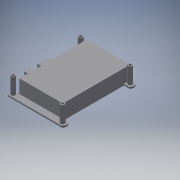
# Autodesk Inventor part: raspberry+touch
Saved by Autodesk Inventor 2019 (Build 230136000, 136)
## iProperties
Created: 2021-11-18
Part Number: raspberry+touch
Material: Generic
Document SubType Name: Modeling
Designer: Pokick
Density: 1 g/cm^3
Appearance: Default
Author: Pokick
Autodesk Inventor part; units mm, degrees
ref_plane "YZ Plane" through (0, 0, 0) normal (1, 0, 0) x (0, 1, 0)
ref_plane "XZ Plane" through (0, 0, 0) normal (0, 1, 0) x (-1, 0, 0)
ref_plane "XY Plane" through (0, 0, 0) normal (0, 0, 1) x (1, 0, 0)
sketch "Sketch1" plane through (0, 0, 0) normal (0, 1, 0) x (-1, 0, 0)
  line L0 (-29.02, 49.29) -> (29.02, 49.29)
  line L1 (29.02, 49.29) -> (29.02, 40.715) construction
  line L2 (29.02, -49.29) -> (-29.02, -49.29)
  line L3 (-29.02, -49.29) -> (-29.02, -40.715) construction
  line L4 (-29.02, 49.29) -> (29.02, -49.29) construction
  line L5 (29.02, 49.29) -> (-29.02, -49.29) construction
  line L6 (-33, 45) -> (33, 45) construction
  line L7 (33, 45) -> (33, -45) construction
  line L8 (33, -45) -> (-33, -45) construction
  line L9 (-33, -45) -> (-33, 45) construction
  line L10 (-33, 45) -> (33, -45) construction
  line L11 (33, 45) -> (-33, -45) construction
  circle A0 centre (33, 45) radius 1.5
  circle A1 centre (33, -45) radius 1.5
  circle A2 centre (-33, -45) radius 1.5
  circle A3 centre (-33, 45) radius 1.5
  line L12 (-38.27, 49.29) -> (38.27, 49.29) construction
  line L13 (38.27, 49.29) -> (38.27, -49.29) construction
  line L14 (38.27, -49.29) -> (-38.27, -49.29) construction
  line L15 (-38.27, -49.29) -> (-38.27, 49.29) construction
  line L16 (-38.27, 49.29) -> (38.27, -49.29) construction
  line L17 (38.27, 49.29) -> (-38.27, -49.29) construction
  line L18 (-38.27, 40.715) -> (29.02, 40.715) construction
  line L19 (38.27, 40.715) -> (38.27, -40.715) construction
  line L20 (38.27, -40.715) -> (-38.27, -40.715) construction
  line L21 (-38.27, -40.715) -> (-38.27, 40.715) construction
  line L22 (-38.27, 40.715) -> (38.27, -40.715) construction
  line L23 (38.27, 40.715) -> (-38.27, -40.715) construction
  line L24 (29.02, 49.29) -> (36.02, 49.29)
  line L25 (29.02, 40.715) -> (36.02, 40.715)
  arc A4 (36.02, 40.715) -> (36.02, 49.29) centre (33.06, 45.0025) ccw
  line L26 (29.02, 40.715) -> (29.02, -40.715)
  line L27 (0, 49.29) -> (0, -49.29) construction
  line L28 (-29.02, 0) -> (29.02, 0) construction
  line L29 (-38.27, -49.29) -> (38.27, -49.29) construction
  line L30 (-38.27, -40.715) -> (38.27, -40.715) construction
  line L31 (29.02, -49.29) -> (36.02, -49.29)
  line L32 (29.02, -40.715) -> (36.02, -40.715)
  arc A5 (36.02, -49.29) -> (36.02, -40.715) centre (33.06, -45.0025) ccw
  line L33 (0, -49.29) -> (0, 49.29) construction
  line L34 (-33, 45) -> (-33, -45) construction
  line L35 (38.27, 49.29) -> (-38.27, 49.29) construction
  line L36 (-38.27, 49.29) -> (-38.27, -49.29) construction
  line L37 (-38.27, -49.29) -> (38.27, -49.29) construction
  line L38 (38.27, 40.715) -> (-38.27, 40.715) construction
  line L39 (-38.27, -40.715) -> (38.27, -40.715) construction
  line L40 (-29.02, 49.29) -> (-36.02, 49.29)
  line L41 (-29.02, 40.715) -> (-36.02, 40.715)
  arc A6 (-36.02, 49.29) -> (-36.02, 40.715) centre (-33.06, 45.0025) ccw
  line L42 (38.27, -49.29) -> (-38.27, -49.29) construction
  line L43 (-29.02, -49.29) -> (-36.02, -49.29)
  line L44 (38.27, -40.715) -> (-38.27, -40.715) construction
  line L45 (-29.02, -40.715) -> (-36.02, -40.715)
  arc A7 (-36.02, -40.715) -> (-36.02, -49.29) centre (-33.06, -45.0025) ccw
  line L46 (-29.02, -40.715) -> (-29.02, 40.715)
  line L47 (-29.02, 40.715) -> (-29.02, 49.29) construction
  line L48 (29.02, 40.715) -> (38.27, 40.715) construction
  line L49 (29.02, -40.715) -> (29.02, -49.29) construction
  point P0 (0, 0)
  dimension "d0" = 58.04
  dimension "d1" = 98.58
  dimension "d2" = 66
  dimension "d3" = 90
  dimension "d4" = 3
  dimension "d5" = 3
  dimension "d6" = 3
  dimension "d7" = 3
  dimension "d8" = 76.54
  dimension "d9" = 98.58
  dimension "d10" = 76.54
  dimension "d11" = 81.43
  dimension "d12" = 7
  dimension "d13" = 7
  constraints: 100 end point, 22 symmetric about line, 17 parallel, 13 point on line, 11 midpoint, 9 perpendicular, 8 centre point, 8 point on circle, 5 horizontal, 4 coincident, 1 tangent, 3 other
  measures "d0" distance of L2.start L2.end
  measures "d1" distance of L0.end L2.start
  measures "d2" distance of L7.end L8.end
  measures "d3" distance of L6.end L7.end
  measures "d4" diameter of A0
  measures "d5" diameter of A1
  measures "d6" diameter of A2
  measures "d7" diameter of A3
  measures "d8" distance of L13.end L14.end
  measures "d9" distance of L12.end L13.end
  measures "d10" distance of L19.end L20.end
  measures "d11" distance of L19.start L19.end
  measures "d12" distance of L0.end L24.end
  measures "d13" distance of L1.end L25.end
extrude "Extrusion1" add sketch "Sketch1" along normal blind 2
sketch "Sketch2" plane through (0, 2, 0) normal (0, 1, 0) x (1, 0, 0)
  line L0 (29.02, -49.29) -> (-29.02, -49.29) construction
  line L1 (-29.02, -49.29) -> (-29.02, 49.29) construction
  line L2 (-29.02, 49.29) -> (29.02, 49.29) construction
  line L3 (29.02, 49.29) -> (29.02, -49.29) construction
  line L4 (29.02, -49.29) -> (-29.02, 49.29) construction
  line L5 (-29.02, -49.29) -> (29.02, 49.29) construction
  line L6 (29.02, 40.715) -> (29.02, -40.715) projected
  line L7 (-29.02, 49.29) -> (29.02, 49.29)
  line L8 (29.02, 49.29) -> (29.02, -40.71)
  line L9 (29.02, -40.71) -> (-29.02, -40.71)
  line L10 (-29.02, -40.71) -> (-29.02, 49.29)
  point P0 (0, 0)
  dimension "d16" = 58.04
  dimension "d17" = 98.58
  dimension "d18" = 90
  constraints: 20 end point, 4 parallel, 2 horizontal, 2 midpoint, 2 perpendicular, 1 point on line
  measures "d16" distance of L1.end L2.end
  measures "d17" distance of L0.end L1.end
  measures "d18" distance of L7.end L8.end
extrude "Extrusion2" add sketch "Sketch2" along normal blind 18
sketch "Sketch3" plane through (-29.02, 0, -40.715) normal (-1, 0, 0) x (0, 0, 1)
  line L0 (-8.575, 0) -> (-8.575, 2) projected
  line L1 (-8.575, 0) -> (37.425, 0) construction
  line L2 (81.43, 0) -> (0, 0) construction
  line L3 (37.425, 0) -> (52.425, 0) construction
  line L4 (37.425, 0) -> (52.425, 0)
  line L5 (52.425, 0) -> (52.425, 20)
  line L6 (52.425, 20) -> (37.425, 20)
  line L7 (37.425, 20) -> (37.425, 0)
  line L8 (81.43, 0) -> (90.005, 0) construction
  line L9 (90.005, 0) -> (70.005, 0) construction
  line L10 (70.005, 0) -> (62.005, 0) construction
  line L11 (62.005, 0) -> (70.005, 0)
  line L12 (70.005, 0) -> (70.005, 20)
  line L13 (70.005, 20) -> (62.005, 20)
  line L14 (62.005, 20) -> (62.005, 0)
  point P0 (40.715, 0)
  dimension "d21" = 46
  dimension "d22" = 15
  dimension "d23" = 20
  dimension "d24" = 15
  dimension "d25" = 20
  dimension "d26" = 8
  dimension "d27" = 8
  dimension "d28" = 20
  constraints: 24 end point, 4 parallel, 4 point on line, 2 horizontal, 2 perpendicular
  measures "d21" distance of L0.start L1.end
  measures "d22" distance of L1.end L3.end
  measures "d23" distance of L5.end L4.end
  measures "d24" distance between parallel lines of L7 L5
  measures "d25" distance of L8.end L9.end
  measures "d26" distance of L9.end L10.end
  measures "d27" distance of L13.end L12.end
  measures "d28" distance of L12.end L11.end
extrude "Extrusion3" add sketch "Sketch3" along normal blind 5
sketch "Sketch5" plane through (0, 0, 0) normal (0, -1, 0) x (1, 0, 0)
  circle A0 centre (-33, 45) radius 1.5 construction
  line L0 (33, -45) -> (-33, -45) construction
  line L1 (-33, -45) -> (-33, 45) construction
  line L2 (-33, 45) -> (33, 45) construction
  line L3 (33, 45) -> (33, -45) construction
  line L4 (33, -45) -> (-33, 45) construction
  line L5 (-33, -45) -> (33, 45) construction
  circle A1 centre (-33, -45) radius 1.5
  circle A2 centre (33, -45) radius 1.5
  circle A3 centre (33, 45) radius 1.5 projected
  circle A4 centre (33, 45) radius 1.5
  circle A5 centre (-33, 45) radius 1.5
  line L6 (-35.5, -43.5566) -> (-33, -42.1132)
  line L7 (-33, -42.1132) -> (-30.5, -43.5566)
  line L8 (-30.5, -43.5566) -> (-30.5, -46.4434)
  line L9 (-30.5, -46.4434) -> (-33, -47.8868)
  line L10 (-33, -47.8868) -> (-35.5, -46.4434)
  line L11 (-35.5, -46.4434) -> (-35.5, -43.5566)
  line L12 (30.5, -43.5566) -> (33, -42.1132)
  line L13 (33, -42.1132) -> (35.5, -43.5566)
  line L14 (35.5, -43.5566) -> (35.5, -46.4434)
  line L15 (35.5, -46.4434) -> (33, -47.8868)
  line L16 (33, -47.8868) -> (30.5, -46.4434)
  line L17 (30.5, -46.4434) -> (30.5, -43.5566)
  line L18 (30.5, 46.4434) -> (33, 47.8868)
  line L19 (33, 47.8868) -> (35.5, 46.4434)
  line L20 (35.5, 46.4434) -> (35.5, 43.5566)
  line L21 (35.5, 43.5566) -> (33, 42.1132)
  line L22 (33, 42.1132) -> (30.5, 43.5566)
  line L23 (30.5, 43.5566) -> (30.5, 46.4434)
  line L24 (-35.5, 46.4434) -> (-33, 47.8868)
  line L25 (-33, 47.8868) -> (-30.5, 46.4434)
  line L26 (-30.5, 46.4434) -> (-30.5, 43.5566)
  line L27 (-30.5, 43.5566) -> (-33, 42.1132)
  line L28 (-33, 42.1132) -> (-35.5, 43.5566)
  line L29 (-35.5, 43.5566) -> (-35.5, 46.4434)
  point P0 (0, 0)
  point P1 (30.5, 45)
  point P2 (-35.5, 45)
  dimension "d31" = 3
  dimension "d32" = 3
  dimension "d33" = 3
  dimension "d34" = 3
  dimension "d35" = 5
  dimension "d36" = 5
  dimension "d37" = 5
  dimension "d38" = 5
  constraints: 60 end point, 8 coincident, 4 centre point, 4 midpoint, 4 parallel, 2 point on line, 1 horizontal, 1 perpendicular, 52 other
  measures "d31" diameter of A1
  measures "d32" diameter of A2
  measures "d33" diameter of A4
  measures "d34" diameter of A5
  measures "d35" distance between parallel lines of L26 L29
  measures "d36" distance between parallel lines of L8 L11
  measures "d37" distance between parallel lines of L17 L14
  measures "d38" distance between parallel lines of L23 L20
extrude "Extrusion4" add sketch "Sketch5" against normal blind 22 from surface at -2
sketch "Sketch6" plane through (0, 0, 0) normal (0, -1, 0) x (1, 0, 0)
  line L0 (-35.8509, -30.6551) -> (-35.8509, -21.9955) construction
  line L1 (-35.8509, -21.9955) -> (-14.7214, -21.9955) construction
  line L2 (-14.7214, -21.9955) -> (-14.7214, -30.6551) construction
  line L3 (-14.7214, -30.6551) -> (-35.8509, -30.6551) construction
  point P0 (0, 0)
  constraints: 2 other
sketch "Sketch7" plane through (36.02, 0, -49.29) normal (0, 0, -1) x (-1, 0, 0)
  line L0 (36.02, 0) -> (63.02, 0) construction
  line L1 (0, 0) -> (72.04, 0) projected
  line L2 (63.02, 0) -> (11.02, 0)
  line L3 (11.02, 0) -> (11.02, 16)
  line L4 (11.02, 16) -> (63.02, 16)
  line L5 (63.02, 16) -> (63.02, 0)
  dimension "d41" = 27
  dimension "d42" = 52
  dimension "d43" = 16
  constraints: 10 end point, 2 parallel, 1 horizontal, 1 perpendicular, 1 point on line
  measures "d41" distance of L0.start L0.end
  measures "d42" distance of L3.end L4.end
  measures "d43" distance of L2.end L3.end
extrude "Extrusion5" add sketch "Sketch7" along normal blind 2
sketch "Sketch8" plane through (0, 0, 0) normal (0, -1, 0) x (1, 0, 0)
  line L0 (-24.9386, -43.252) -> (-24.9386, 42.092) construction
  line L1 (-24.9386, 42.092) -> (23.0674, 42.092) construction
  line L2 (23.0674, 42.092) -> (23.0674, -43.252) construction
  line L3 (23.0674, -43.252) -> (-24.9386, -43.252) construction
  point P0 (0, 0)
  constraints: 2 other
equation "\"d24\" = d22"
body "Solid1"
